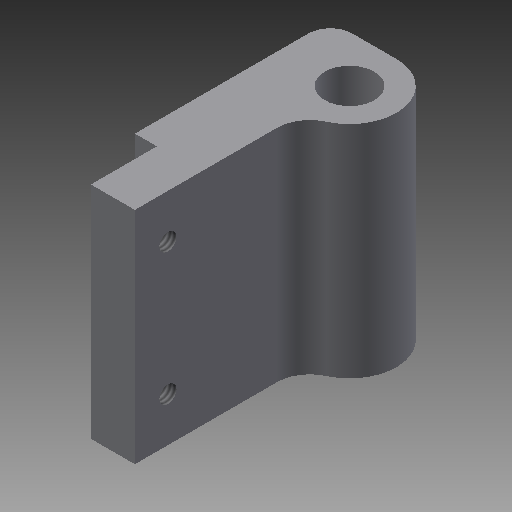
# Autodesk Inventor part: Türarm
Saved by Autodesk Inventor 2018 (Build 220112000, 112)
## iProperties
Created: 2013-02-19
Part Number: Türarm
Material: Generic
Document SubType Name: Modeling
Designer: Neef
Density: 1 g/cm^3
Appearance: Default
Author: Neef
Autodesk Inventor part; units mm, degrees
note: some values were not read from the file. Chosen so that the rebuilt part matches the saved one: direction of "Bohrung1"; direction of "Bohrung2".
ref_plane "YZ Plane" through (0, 0, 0) normal (1, 0, 0) x (0, 1, 0)
ref_plane "XZ Plane" through (0, 0, 0) normal (0, 1, 0) x (-1, 0, 0)
ref_plane "XY Plane" through (0, 0, 0) normal (0, 0, 1) x (1, 0, 0)
sketch "Skizze1" plane through (0, 0, 0) normal (0, 0, 1) x (1, 0, 0)
  circle A0 centre (0, 0) radius 2.25
  line L0 (0, 4.25) -> (-6, 4.25)
  line L1 (-6, 4.25) -> (-6, -13.5)
  line L2 (-6, -13.5) -> (-4, -13.5)
  line L3 (-4, -13.5) -> (-4, -19.5)
  line L4 (-4, -19.5) -> (0, -19.5)
  line L5 (0, -19.5) -> (0, -4.25)
  arc A1 (0, -4.25) -> (0, 4.25) centre (0, 0) ccw
  line L6 (0, 9) -> (0, -24.25) projected
  line L7 (-8.05, 0) -> (6.3, 0) projected
  dimension "d0" = 4.5
  dimension "d1" = 4
  dimension "d2" = 2
  dimension "d3" = 2
  dimension "d4" = 13.5
  dimension "d5" = 6
  constraints: 12 end point, 4 parallel, 2 centre point, 2 coincident, 2 point on circle, 1 collinear, 1 horizontal, 1 perpendicular, 1 point on line
  measures "d0" diameter of A0
  measures "d1" distance of L3.end L4.end
  measures "d2" distance of L1.end L2.end
  measures "d3" radial gap between concentric circles of A0 A1
  measures "d4" distance from line of point (0, 0) L2
  measures "d5" distance of L2.end L3.end
extrude "Extrusion1" add sketch "Skizze1" along normal blind 20 contours L7 A1 L6 A0 | A0 L6 A1 L7 | A0 L7 L1 L0 L6 | L6 L5 L4 L3 L2 L1 L7 A0
sketch "Skizze2" plane through (-6, -13.5, 0) normal (-1, 0, 0) x (0, 0, 1)
  line L0 (20, 0) -> (20, 17.75) projected
  line L1 (0, 17.75) -> (0, 0) projected
  line L2 (0, 15.75) -> (20, 15.75) projected
  line L3 (0, 11.25) -> (20, 11.25) projected
  point P0 (0, 13.5)
  point P1 (4, 13.5)
  point P2 (16, 13.5)
  dimension "d8" = 4
  dimension "d9" = 4
  measures "d8" distance from line of L1 point (4, 13.5)
  measures "d9" distance from line of L0 point (16, 13.5)
hole "Bohrung1" at (-6, 0, 4) at (-6, 0, 16) direction (1, 0, 0) diameter 1.567 end up to surface thread size "M2x0.4" class "6H" standard "ISO Metric profile"
sketch "Skizze3" plane through (-4, -19.5, 0) normal (-1, 0, 0) x (0, 0, 1)
  line L0 (20, 0) -> (20, 6) projected
  line L1 (0, 6) -> (0, 0) projected
  point P0 (0, 19.5)
  point P1 (4, 3)
  point P2 (16, 3)
  dimension "d17" = 4
  dimension "d18" = 4
  measures "d17" distance from line of L1 point (4, 3)
  measures "d18" distance from line of L0 point (16, 3)
hole "Bohrung2" at (-4, -16.5, 4) at (-4, -16.5, 16) direction (1, 0, 0) diameter 1.567 end up to surface thread size "M2x0.4" class "6H" standard "ISO Metric profile"
fillet "Rundung1" radius 2 1 edges at (-6, 4.25, 10)
fillet "Rundung2" radius 3 1 edges at (0, -4.25, 10)
equation "\"d9\" = d8"
equation "\"d18\" = d17"
